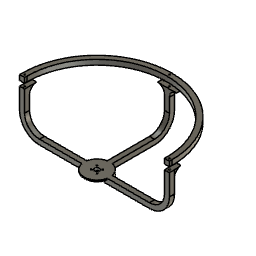
symmetrical_propeller_guard v12 (Autodesk Fusion 360 design; units mm, degrees)
Autodesk Fusion 360 part; units mm, degrees
sketch "Sketch1" plane through (0, 0, 0) normal (0, 0, 1) x (1, 0, 0)
  circle A0 centre (0, 0) radius 26
  dimension "d1" = 52
  constraint coincident A0.centre origin
  measures "d1" diameter of A0
extrude "Extrude1" add sketch "Sketch1" along normal blind 10 makes body 1
sketch "Sketch2" plane through (0, 0, 0) normal (0, 1, 0) x (1, 0, 0)
  line L0 (0, 0) -> (110, 0)
  arc A0 (150, -40) -> (110, 0) centre (110, -40) ccw
  line L1 (150, -40) -> (150, -82)
  line L2 (150, -82) -> (140, -82)
  arc A1 (140, -40) -> (110, -10) centre (110, -40) ccw
  line L3 (140, -82) -> (140, -40)
  line L4 (110, -10) -> (0, -10)
  line L5 (0, -10) -> (0, 0)
  dimension "d4" = 110
  dimension "d5" = 110
  dimension "d6" = 10
  dimension "d7" = 30
  dimension "d8" = 40
  dimension "d9" = 10
  dimension "d40" = 42
  constraint coincident L0.start L5.end
  constraint horizontal L0
  constraint tangent A0 L1
  constraint vertical L1
  constraint perpendicular L1 L2
  constraint coincident A0.centre A1.centre
  constraint tangent A1 L3
  constraint tangent A1 L4
  constraint perpendicular L3 L4
  constraint perpendicular L0 L5
  measures "d4" distance of L0.start L0.end
  measures "d5" distance of A1.end L4.end
  measures "d6" distance of L4.end L0.start
  measures "d7" radius of A1
  measures "d8" radius of A0
  measures "d9" distance of L1.end L2.end
  measures "d40" distance of A0.start L1.end
extrude "Extrude2" add sketch "Sketch2" along normal mid plane 10 bodies 1
pattern_circular "C-Pattern1" count 3 over 180 about axis through (0, 0, 1.75) along (0, 0, 1) of "Extrude2"
sketch "Sketch3" plane through (0, 0, 82) normal (0, 0, 1) x (-1, 0, 0)
  line L0 (-150, 5) -> (-150, -5)
  line L1 (-150, -5) -> (-140, -5)
  line L2 (-140, -5) -> (-140, 5)
  line L3 (-140, 5) -> (-150, 5)
  arc A0 (-140, 0) -> (140, 0) centre (0, 0) ccw
  arc A1 (-150, 0) -> (150, 0) centre (0, 0) ccw
  line L4 (150, 0) -> (150, 5)
  line L5 (150, 5) -> (140, 5)
  line L6 (140, 5) -> (140, 0)
  line L7 (-150, 0) -> (-150, 5)
  line L8 (-140, 5) -> (-140, 0)
  constraint tangent L2 A0
  constraint tangent L0 A1
  constraint tangent A1 L4
  constraint vertical L4
  constraint perpendicular L4 L5
  constraint tangent A0 L6
  constraint coincident L0.start L3.end
  constraint tangent A1 L7
  constraint coincident L2.end L3.start
  constraint tangent A0 L8
extrude "Extrude3" add sketch "Sketch3" along normal blind 10 contours L0 L1 L2 L3 A1 L7 L8 | L1 L2 A0 A1 L4 L5 L6 bodies 1
fillet "Fillet1" chord length 20 4 edges at (144.9583, 5, 82) (5, 144.9583, 82) (-144.9583, 5, 82) (-5, 144.9583, 82) on bodies 1
sketch "Sketch4" plane through (0, 0, 0) normal (0, 0, -1) x (1, 0, 0)
  arc A0 (-25.5147, -5) -> (-5, -25.5147) centre (0, 0) ccw
  line L0 (-5, -25.5147) -> (-5, -110)
  line L1 (-5, -110) -> (5, -110)
  line L2 (5, -110) -> (5, -25.5147)
  arc A1 (5, -25.5147) -> (25.5147, -5) centre (0, 0) ccw
  line L3 (25.5147, -5) -> (110, -5)
  line L4 (110, -5) -> (110, 5)
  line L5 (110, 5) -> (25.5147, 5)
  arc A2 (25.5147, 5) -> (-25.5147, 5) centre (0, 0) ccw
  line L6 (-25.5147, 5) -> (-110, 5)
  line L7 (-110, 5) -> (-110, -5)
  line L8 (-110, -5) -> (-25.5147, -5)
  circle A3 centre (0, 0) radius 20.5
  line L9 (-30, 30) -> (30, 30)
  line L10 (30, 30) -> (30, 5)
  line L11 (30, 5) -> (-30, 5)
  line L12 (-30, 5) -> (-30, 30)
  dimension "d39" = 41
  constraint concentric A0 A3
  constraint horizontal L9
  constraint vertical L10
  constraint horizontal L11
  constraint vertical L12
  constraint coincident L5 L10.end
  measures "d39" diameter of A3
extrude "Extrude5" cut sketch "Sketch4" against normal blind 5 contours L5 A2 L6 L9 L10 L11 L12 | A2 A3 L11 | A3 L11 | A3 L11 bodies 1
chamfer "Chamfer1" distance 3 angle 45 1 edges at (0, -26, 5) on bodies 1
sketch "Sketch5" plane through (0, 0, 10) normal (0, 0, 1) x (-1, 0, 0)
  arc A0 (25.5147, 5) -> (-25.5147, 5) centre (0, 0) ccw
  line L0 (-25.5147, 5) -> (-110, 5)
  line L1 (-110, 5) -> (-110, -5)
  line L2 (-110, -5) -> (-25.5147, -5)
  arc A1 (-25.5147, -5) -> (-5, -25.5147) centre (0, 0) ccw
  line L3 (-5, -25.5147) -> (-5, -110)
  line L4 (-5, -110) -> (5, -110)
  line L5 (5, -110) -> (5, -25.5147)
  arc A2 (5, -25.5147) -> (25.5147, -5) centre (0, 0) ccw
  line L6 (25.5147, -5) -> (110, -5)
  line L7 (110, -5) -> (110, 5)
  line L8 (110, 5) -> (25.5147, 5)
  circle A3 centre (0, 0) radius 5
  circle A4 centre (-5.6569, -5.6569) radius 1.5
  circle A5 centre (6.7175, -6.7175) radius 1.5
  circle A6 centre (5.6569, 5.6569) radius 1.5
  circle A7 centre (-6.7175, 6.7175) radius 1.5
  dimension "d26" = 10
  dimension "d27" = 3
  dimension "d28" = 3
  dimension "d29" = 8
  dimension "d30" = 9.5
  dimension "d31" = 6.7175
  dimension "d32" = 5.6569
  dimension "d34" = 360
  constraint coincident A0.centre A1.centre
  measures "d26" diameter of A3
  measures "d27" diameter of A4
  measures "d28" diameter of A5
  measures "d29" distance of A0.centre A4.centre
  measures "d30" distance of A0.centre A5.centre
  measures "d31" horizontal distance of A0.centre A5.centre
  measures "d32" horizontal distance of A0.centre A4.centre
extrude "Extrude6" cut sketch "Sketch5" against normal blind 5 contours A3 | A4 | A5 | A6 | A7 bodies 1
sketch "Sketch7" plane through (0, 0, 92) normal (0, 0, 1) x (-1, 0, 0)
  line L0 (149.9166, -5) -> (150, -5)
  line L1 (150, 5) -> (140, 5)
  line L2 (140, 5) -> (140, -19.1421)
  circle A0 centre (145, 0) radius 1.5
  circle A1 centre (-145, 0) radius 1.5
  circle A2 centre (0, -145) radius 1.5
  line L3 (-150, 5) -> (-150, -5)
  line L4 (-150, 5) -> (-140, 5)
  line L5 (150, -5) -> (150, 5)
  line L6 (148.7736, -19.1421) -> (140, -19.1421)
  arc A3 (148.7736, -19.1421) -> (149.9166, -5) centre (0, 0) ccw
  arc A4 (-150, 0) -> (150, 0) centre (0, 0) ccw
  line L7 (150, 0) -> (150, 5)
  line L8 (150, 5) -> (140, 5)
  line L9 (140, 5) -> (140, 0)
  arc A5 (-140, 0) -> (140, 0) centre (0, 0) ccw
  line L10 (-140, 0) -> (-140, 5)
  line L11 (-140, 5) -> (-150, 5)
  line L12 (-150, 5) -> (-150, 0)
  dimension "d43" = 3
  dimension "d44" = 5
  dimension "d45" = 5
  dimension "d46" = 3
  dimension "d47" = 5
  dimension "d48" = 5
  dimension "d49" = 3
  measures "d43" diameter of A0
  measures "d44" distance of L2 A0.centre
  measures "d45" distance of L1 A0.centre
  measures "d46" diameter of A1
  measures "d47" distance of A1.centre L3
  measures "d48" distance of A1.centre L4
  measures "d49" diameter of A2
hole "Hole1" at (0, 145, 92) at (-145, 0, 92) at (145, 0, 92) direction (0, 0, -1) diameter 3 depth 10 tip angle 118 bodies 1
ref_plane "WorkPlane1" through (0, 0, 82) normal (0, 0, 1) x (1, 0, 0)
split "Split1" by plane through (0, 0, 82) normal (0, 0, 1) bodies 1 makes body 2 at (0, 150, 88.6667)
move_body "Move3" bodies 2 to x (1, 0, 0) y (0, 1, 0) z (0, 0, 1) at (0, 0, 10)
